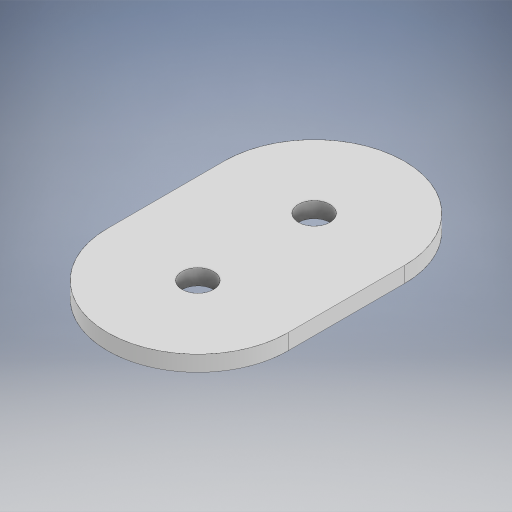
# Autodesk Inventor part: circle
Saved by Autodesk Inventor 2024 (Build 280153000, 153)
## iProperties
Created: 2024-12-18
Part Number: circle
Material: Generic
Document SubType Name: Modeling
Designer: Alex
Density: 1 g/cm^3
Appearance: Default
Author: Alex
Autodesk Inventor part; units mm, degrees
ref_plane "YZ Plane" through (0, 0, 0) normal (1, 0, 0) x (0, 1, 0)
ref_plane "XZ Plane" through (0, 0, 0) normal (0, 1, 0) x (-1, 0, 0)
ref_plane "XY Plane" through (0, 0, 0) normal (0, 0, 1) x (1, 0, 0)
sketch "Sketch1" plane through (0, 0, 0) normal (0, 1, 0) x (-1, 0, 0)
  line L0 (0, 0) -> (-40.16, 0) construction
  line L1 (-40.16, 0) -> (-40.16, -66.05) construction
  line L2 (-40.16, -66.05) -> (0, -66.05) construction
  line L3 (0, -66.05) -> (0, 0) construction
  circle A0 centre (-20.08, -20.08) radius 20.08 construction
  circle A1 centre (-20.08, -45.97) radius 20.08 construction
  arc A2 (0, -20.08) -> (-40.16, -20.08) centre (-20.08, -20.08) ccw
  arc A3 (-40.16, -45.97) -> (0, -45.97) centre (-20.08, -45.97) ccw
  line L4 (0, -20.08) -> (0, -45.97)
  line L5 (-40.16, -45.97) -> (-40.16, -20.08)
  circle A4 centre (-20.08, -45.97) radius 3.5
  circle A5 centre (-20.08, -20.08) radius 3.5
  dimension "d0" = 40.16
  dimension "d1" = 66.05
  dimension "d2" = 7
  dimension "d3" = 7
  constraints: 12 end point, 10 tangent, 8 point on circle, 6 centre point, 4 point on line, 2 coincident, 2 parallel, 1 collinear, 1 horizontal, 1 perpendicular
  measures "d0" distance of L2.end L1.end
  measures "d1" distance of L1.end L0.end
  measures "d2" diameter of A4
  measures "d3" diameter of A5
extrude "Extrusion1" add sketch "Sketch1" along normal blind 3.5
body "Solid1"
